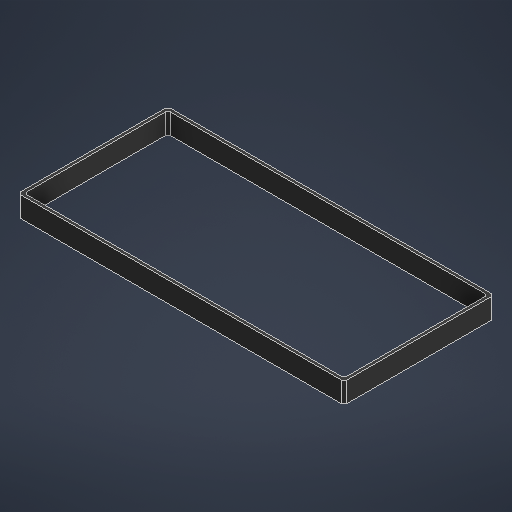
# Autodesk Inventor part: band 18t
Saved by Autodesk Inventor 2025.2 (Build 292293000, 293)
## iProperties
Created: 2026-01-02
Part Number: band 18t
Material: Rubber
Document SubType Name: Modeling
Designer: cloudy
Density: 0.93 g/cm^3
Appearance: Rubber - Black
Author: cloudy
Autodesk Inventor part; units mm, degrees
ref_plane "YZ Plane" through (0, 0, 0) normal (1, 0, 0) x (0, 1, 0)
ref_plane "XZ Plane" through (0, 0, 0) normal (0, 1, 0) x (-1, 0, 0)
ref_plane "XY Plane" through (0, 0, 0) normal (0, 0, 1) x (1, 0, 0)
sketch "Sketch1" plane through (0, 0, 0) normal (0, 1, 0) x (-1, 0, 0)
  line L0 (49.53, 22.225) -> (-49.53, 22.225)
  line L1 (-49.53, 22.225) -> (-49.53, -22.225)
  line L2 (-49.53, -22.225) -> (49.53, -22.225)
  line L3 (49.53, -22.225) -> (49.53, 22.225)
  line L4 (49.53, 22.225) -> (-49.53, -22.225) construction
  line L5 (-49.53, 22.225) -> (49.53, -22.225) construction
  line L6 (50.53, 23.225) -> (-50.53, 23.225)
  line L7 (-50.53, 23.225) -> (-50.53, -23.225)
  line L8 (-50.53, -23.225) -> (50.53, -23.225)
  line L9 (50.53, -23.225) -> (50.53, 23.225)
  point P0 (0, 0)
  dimension "d0" = 44.45
  dimension "d1" = 99.06
  dimension "d2" = 1
  constraints: 20 end point, 4 parallel, 2 midpoint, 2 perpendicular, 1 horizontal, 3 other
  measures "d0" distance of L0.end L1.end
  measures "d1" distance of L1.end L2.end
  measures "d2" distance between parallel lines of L3 L9
extrude "Extrusion1" add sketch "Sketch1" along normal blind 6.35
chamfer "Chamfer1" distance 0.7937 angle 45 8 edges at (-50.53, 3.175, -23.225) (-49.53, 3.175, -22.225) (-49.53, 3.175, 22.225) (-50.53, 3.175, 23.225) (50.53, 3.175, -23.225) (49.53, 3.175, -22.225) (49.53, 3.175, 22.225) (50.53, 3.175, 23.225)
body "Solid1"
